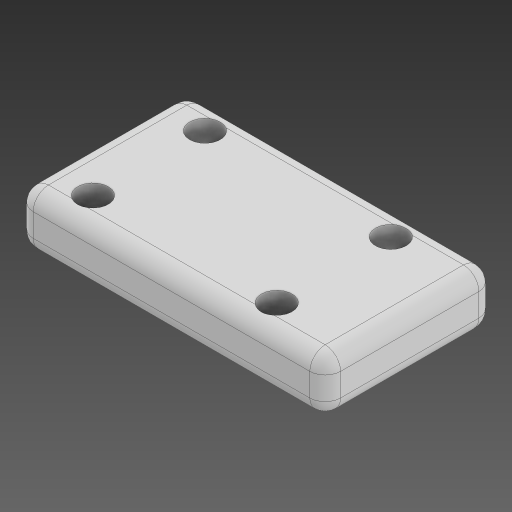
# Autodesk Inventor part: Деталь3
Saved by Autodesk Inventor 2023 (Build 270158000, 158)
## iProperties
Created: 2025-06-23
Part Number: Деталь3
Material: Типовые
Document SubType Name: Modeling
Designer: daa
Density: 1 g/cm^3
Appearance: По умолчанию
Author: daa
Autodesk Inventor part; units mm, degrees
ref_plane "YZ Plane" through (0, 0, 0) normal (1, 0, 0) x (0, 1, 0)
ref_plane "XZ Plane" through (0, 0, 0) normal (0, 1, 0) x (-1, 0, 0)
ref_plane "XY Plane" through (0, 0, 0) normal (0, 0, 1) x (1, 0, 0)
sketch "Эскиз1" plane through (0, 0, 0) normal (0, 1, 0) x (-1, 0, 0)
  line L0 (40, 22) -> (0, 22)
  line L1 (0, 22) -> (0, 0)
  line L2 (0, 0) -> (40, 0)
  line L3 (40, 0) -> (40, 22)
  circle A0 centre (33.9283, 18.2892) radius 2
  circle A1 centre (33.9283, 3.7108) radius 2
  circle A2 centre (9.8763, 18.4209) radius 2
  circle A3 centre (9.8763, 3.5791) radius 2
  dimension "d0" = 40
  dimension "d1" = 22
  dimension "d2" = 4
  dimension "d3" = 4
  dimension "d4" = 4
  dimension "d5" = 4
  dimension "d6" = 6.0717
  dimension "d7" = 6.0717
  dimension "d8" = 3.7108
  dimension "d9" = 3.7108
  dimension "d10" = 9.8763
  dimension "d11" = 9.8763
  dimension "d12" = 3.5791
  dimension "d13" = 3.5791
  constraints: 8 end point, 4 centre point, 2 parallel, 1 coincident, 1 horizontal, 1 perpendicular
  measures "d0" distance of L2.end L1.end
  measures "d1" distance of L1.end L0.end
  measures "d2" diameter of A0
  measures "d3" diameter of A1
  measures "d4" diameter of A2
  measures "d5" diameter of A3
  measures "d6" distance from line of L3 A0.centre
  measures "d7" distance from line of L3 A1.centre
  measures "d8" distance from line of A0.centre L0
  measures "d9" distance from line of L2 A1.centre
  measures "d10" distance from line of L1 A3.centre
  measures "d11" distance from line of L1 A2.centre
  measures "d12" distance from line of L2 A3.centre
  measures "d13" distance from line of A2.centre L0
extrude "Выдавливание1" add sketch "Эскиз1" along normal blind 7
fillet "Сопряжение1" radius 2 12 edges at (0, 3.5, 22) (0, 3.5, 0) (-40, 3.5, 0) (-40, 3.5, 22) (-40, 0, 11) (-40, 7, 11) (-20, 0, 22) (-20, 7, 22) (0, 0, 11) (0, 7, 11) (-20, 0, 0) (-20, 7, 0)
